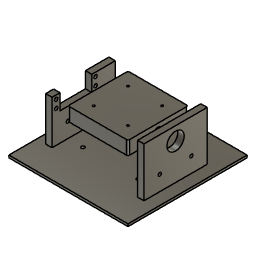
lidar_mount_prototype (Autodesk Fusion 360 design; units mm, degrees)
Autodesk Fusion 360 part; units mm, degrees
sketch "sketchBase" plane through (0, 0, 0) normal (0, 0, 1) x (1, 0, 0)
  line L0 (27.8, 27.8) -> (-27.8, 27.8) construction
  line L1 (-27.8, 27.8) -> (-27.8, -27.8) construction
  line L2 (-27.8, -27.8) -> (27.8, -27.8) construction
  line L3 (27.8, -27.8) -> (27.8, 27.8) construction
  line L4 (27.8, 27.8) -> (-27.8, -27.8) construction
  line L5 (-27.8, 27.8) -> (27.8, -27.8) construction
  line L6 (37.8, 37.8) -> (-37.8, 37.8) construction
  line L7 (-37.8, 37.8) -> (-37.8, -37.8) construction
  line L8 (-37.8, -37.8) -> (37.8, -37.8) construction
  line L9 (37.8, -37.8) -> (37.8, 37.8) construction
  line L10 (37.8, 37.8) -> (-37.8, -37.8) construction
  line L11 (-37.8, 37.8) -> (37.8, -37.8) construction
  line L12 (75, 75) -> (-75, 75)
  line L13 (-75, 75) -> (-75, -75)
  line L14 (-75, -75) -> (75, -75)
  line L15 (75, -75) -> (75, 75)
  line L16 (75, 75) -> (-75, -75) construction
  line L17 (-75, 75) -> (75, -75) construction
  line L18 (-55.8, 39.8) -> (-63.8, 39.8) construction
  line L19 (-63.8, 39.8) -> (-63.8, -39.8) construction
  line L20 (-63.8, -39.8) -> (-55.8, -39.8) construction
  line L21 (-55.8, -39.8) -> (-55.8, 39.8) construction
  line L22 (-55.8, 39.8) -> (-63.8, -39.8) construction
  line L23 (-63.8, 39.8) -> (-55.8, -39.8) construction
  line L24 (59.9, -39.8) -> (59.9, 39.8) construction
  line L25 (59.9, -39.8) -> (51.9, 39.8) construction
  line L26 (51.9, -39.8) -> (59.9, 39.8) construction
  line L27 (51.9, 39.8) -> (51.9, -39.8) construction
  line L28 (51.9, -39.8) -> (59.9, -39.8) construction
  line L29 (59.9, 39.8) -> (51.9, 39.8) construction
  line L30 (-37.8, 0) -> (-36.8, 0) construction
  line L31 (37.8, 0) -> (42.8, 0) construction
  line L32 (42.8, 0) -> (50.8, 0) construction
  line L33 (50.8, 0) -> (52.4, 0) construction
  line L34 (52.4, 0) -> (59.4, 0) construction
  line L35 (59.4, 0) -> (59.9, 0) construction
  line L36 (59.9, 0) -> (55.9, 0) construction
  line L37 (51.9, 0) -> (51.9, -19.9) construction
  line L38 (51.9, -19.9) -> (32.9, -19.9) construction
  circle A0 centre (-36.8, -19.9) radius 2 construction
  circle A1 centre (-36.8, -19.9) radius 2.1
  circle A2 centre (-36.8, 19.9) radius 2.1
  circle A3 centre (-36.8, 19.9) radius 2 construction
  circle A4 centre (32.9, -19.9) radius 2 construction
  circle A5 centre (32.9, -19.9) radius 2.1
  circle A6 centre (32.9, 19.9) radius 2 construction
  circle A7 centre (32.9, 19.9) radius 2.1
  line L39 (-36.8, 0) -> (-43.3, 0) construction
  line L40 (-43.3, 0) -> (-55.8, 0) construction
  line L41 (-55.8, 0) -> (-55.8, -19.9) construction
  line L42 (-55.8, -19.9) -> (-36.8, -19.9) construction
  point P0 (-59.8, 0)
  point P1 (55.9, 0)
  dimension "d93" = 55.6
  dimension "d94" = 55.6
  dimension "d95" = 75.6
  dimension "d96" = 75.6
  dimension "d99" = 150
  dimension "d100" = 150
  dimension "d109" = 8
  dimension "d110" = 79.6
  dimension "d307" = 1
  dimension "d344" = 5
  dimension "d345" = 8
  dimension "d346" = 1.6
  dimension "d347" = 7
  dimension "d348" = 0.5
  dimension "d349" = 4
  dimension "d350" = 19.9
  dimension "d351" = 19
  dimension "d358" = 4
  dimension "d359" = 0.1
  dimension "d362" = 0
  dimension "d363" = 39.8
  dimension "d369" = 4
  dimension "d370" = 0.1
  dimension "d373" = 0
  dimension "d374" = 39.8
  dimension "d375" = 6.5
  dimension "d376" = 12.5
  dimension "d377" = 19.9
  dimension "d378" = 19
  constraint horizontal L0
  constraint perpendicular L0 L1
  constraint parallel L0 L2
  constraint parallel L1 L3
  constraint coincident L4 origin
  constraint coincident L5 origin
  constraint horizontal L6
  constraint perpendicular L6 L7
  constraint parallel L6 L8
  constraint coincident L10 origin
  constraint coincident L11 origin
  constraint horizontal L12
  constraint perpendicular L12 L13
  constraint parallel L12 L14
  constraint parallel L13 L15
  constraint coincident L16 origin
  constraint coincident L17 origin
  constraint horizontal L18
  constraint perpendicular L18 L19
  constraint parallel L18 L20
  constraint parallel L19 L21
  constraint coincident L22 P0
  constraint coincident L23 P0
  constraint midpoint L7 L30.start
  constraint perpendicular L7 L30
  constraint midpoint L9 L31.start
  constraint perpendicular L9 L31
  constraint parallel L31 L32
  constraint parallel L32 L33
  constraint perpendicular L24 L34
  constraint parallel L34 L35
  constraint parallel L34 L36
  constraint midpoint L26 P1
  constraint coincident P1 L36.end
  constraint midpoint L27 L37.start
  constraint perpendicular L33 L37
  constraint perpendicular L27 L38
  constraint coincident L38.end A4.centre
  constraint perpendicular L7 L39
  constraint parallel L39 L40
  constraint coincident L21 L40.end
  constraint perpendicular L40 L41
  constraint perpendicular L41 L42
  constraint coincident A0.centre A1.centre
  measures "d93" distance of L1.end L2.end
  measures "d94" distance of L0.end L1.end
  measures "d95" distance of L7.end L8.end
  measures "d96" distance of L6.end L7.end
  measures "d99" distance of L13.end L14.end
  measures "d100" distance of L12.end L13.end
  measures "d109" distance of L19.end L20.end
  measures "d110" distance of L18.end L19.end
  measures "d307" distance of L30.start L30.end
  measures "d344" distance of L31.start L31.end
  measures "d345" distance of L31.end L32.end
  measures "d346" distance of L32.end L33.end
  measures "d347" distance of L33.end L34.end
  measures "d348" distance of L34.end L35.end
  measures "d349" distance of L35.end P1
  measures "d350" distance of L37.start L37.end
  measures "d351" distance of L37.end L38.end
  measures "d358" diameter of A0
  measures "d369" diameter of A4
  measures "d375" distance of L30.end L39.end
  measures "d376" distance of L39.end L40.end
  measures "d377" distance of L40.end L41.end
  measures "d378" distance of L41.end A0.centre
ref_plane "WorkPlane1" through (0, 0, 3) normal (0, 0, 1) x (1, 0, 0)
sketch "sketchSups" plane through (0, 0, 3) normal (0, 0, 1) x (1, 0, 0)
  line L0 (-55.8, 39.8) -> (-63.8, 39.8)
  line L1 (-55.8, -39.8) -> (-55.8, 39.8)
  line L2 (-63.8, 39.8) -> (-63.8, -39.8)
  line L3 (-63.8, -39.8) -> (-55.8, -39.8)
  line L4 (51.9, 39.8) -> (51.9, -39.8)
  line L5 (59.9, 39.8) -> (51.9, 39.8)
  line L6 (59.9, -39.8) -> (59.9, 39.8)
  line L7 (51.9, -39.8) -> (59.9, -39.8)
extrude "Extrude5" add sketch "sketchSups" along normal blind 55 contours L0 L1 L2 L3 makes body 1
extrude "Extrude6" add sketch "sketchSups" along normal blind 62 separate body contours L4 L5 L6 L7 makes body 2
sketch "sketchServoSup" plane through (-55.8, 0, 0) normal (1, 0, 0) x (0, 1, 0)
  line L0 (-39.8, 3) -> (39.8, 3)
  line L1 (39.8, 3) -> (39.8, 58)
  line L2 (39.8, 58) -> (-39.8, 58)
  line L3 (-39.8, 58) -> (-39.8, 3)
  line L4 (0, 58) -> (0, 48.2) construction
  line L5 (0, 48.2) -> (-9.8, 48.2) construction
  line L6 (10, 58) -> (-29.6, 58) construction
  line L7 (-29.6, 58) -> (-29.6, 38.4) construction
  line L8 (-29.6, 38.4) -> (10, 38.4) construction
  line L9 (10, 38.4) -> (10, 58) construction
  line L10 (10, 58) -> (-29.6, 38.4) construction
  line L11 (-29.6, 58) -> (10, 38.4) construction
  line L12 (-9.8, 48.2) -> (-34.55, 48.2) construction
  line L13 (-34.55, 48.2) -> (-34.55, 43.2) construction
  circle A0 centre (-34.55, 43.2) radius 2.05
  circle A1 centre (-34.55, 43.2) radius 2.15
  circle A2 centre (14.95, 43.2) radius 2.15
  circle A3 centre (14.95, 43.2) radius 2.05
  circle A4 centre (-34.55, 53.2) radius 2.15
  circle A5 centre (-34.55, 53.2) radius 2.05
  circle A6 centre (14.95, 53.2) radius 2.15
  circle A7 centre (14.95, 53.2) radius 2.05
  line L14 (0, 3) -> (0, 22) construction
  line L15 (0, 22) -> (-19.9, 22) construction
  circle A8 centre (-19.9, 22) radius 2
  circle A9 centre (-19.9, 22) radius 2.1
  circle A10 centre (19.9, 22) radius 2.1
  circle A11 centre (19.9, 22) radius 2
  line L16 (10.2, 58.2) -> (-29.8, 58.2)
  line L17 (-29.8, 58.2) -> (-29.8, 38.2)
  line L18 (-29.8, 38.2) -> (10.2, 38.2)
  line L19 (10.2, 38.2) -> (10.2, 58.2)
  point P0 (-9.8, 48.2)
  dimension "d147" = 9.8
  dimension "d148" = 9.8
  dimension "d149" = 39.6
  dimension "d150" = 19.6
  dimension "d152" = 24.75
  dimension "d153" = 5
  dimension "d154" = 4.1
  dimension "d155" = 0.1
  dimension "d158" = 49.5
  dimension "d159" = 10
  dimension "d213" = 19
  dimension "d214" = 19.9
  dimension "d215" = 4
  dimension "d216" = 0.1
  dimension "d219" = 39.8
  dimension "d220" = 0
  dimension "d380" = 0.2
  constraint midpoint L2 L4.start
  constraint perpendicular L2 L4
  constraint perpendicular L4 L5
  constraint horizontal L6
  constraint perpendicular L6 L7
  constraint parallel L6 L8
  constraint parallel L7 L9
  constraint coincident L10 P0
  constraint coincident L11 P0
  constraint coincident P0 L5.end
  constraint parallel L5 L12
  constraint perpendicular L12 L13
  constraint coincident L13.end A0.centre
  constraint midpoint L0 L14.start
  constraint perpendicular L0 L14
  constraint perpendicular L14 L15
  constraint coincident L15.end A8.centre
  measures "d147" distance of L4.start L4.end
  measures "d148" distance of L4.end P0
  measures "d149" distance of L7.end L8.end
  measures "d150" distance of L6.end L7.end
  measures "d152" distance of P0 L12.end
  measures "d153" distance of L12.end L13.end
  measures "d154" diameter of A0
  measures "d213" distance of L14.start L14.end
  measures "d214" distance of L14.end L15.end
  measures "d215" diameter of A8
sketch "sketchBearingSup" plane through (51.9, 0, 0) normal (-1, 0, 0) x (0, -1, 0)
  line L0 (-39.8, 3) -> (39.8, 3)
  line L1 (39.8, 3) -> (39.8, 65)
  line L2 (39.8, 65) -> (-39.8, 65)
  line L3 (-39.8, 65) -> (-39.8, 3)
  line L4 (0, 3) -> (0, 22) construction
  line L5 (0, 22) -> (-19.9, 22) construction
  circle A0 centre (-19.9, 22) radius 2
  circle A1 centre (-19.9, 22) radius 2.1
  circle A2 centre (19.9, 22) radius 2
  circle A3 centre (19.9, 22) radius 2.1
  line L6 (0, 3) -> (0, 48.2) construction
  circle A4 centre (0, 48.2) radius 11 construction
  circle A5 centre (0, 48.2) radius 10.85
  circle A6 centre (0, 48.2) radius 3
  line L7 (0, 3) -> (0, 22) construction
  dimension "d223" = 19.9
  dimension "d225" = 4
  dimension "d226" = 0.1
  dimension "d229" = 39.8
  dimension "d230" = 0
  dimension "d252" = 45.2
  dimension "d253" = 22
  dimension "d255" = 0.15
  dimension "d263" = 6
  dimension "d342" = 19
  constraint midpoint L0 L4.start
  constraint perpendicular L0 L4
  constraint perpendicular L4 L5
  constraint coincident L5.end A0.centre
  constraint perpendicular L0 L6
  constraint coincident L6.end A4.centre
  constraint perpendicular L5 L7
  constraint coincident L4.end L5.start
  measures "d223" distance of L4.end L5.end
  measures "d225" diameter of A0
  measures "d252" distance of L4.start L6.end
  measures "d253" diameter of A4
  measures "d263" diameter of A6
  measures "d342" distance of L4.start L4.end
ref_plane "WorkPlane6" through (0, 0, 39.7) normal (0, 0, 1) x (1, 0, 0)
sketch "sketchLidarSup" plane through (0, 0, 39.7) normal (0, 0, 1) x (1, 0, 0)
  line L0 (-37.8, 37.8) -> (-37.8, -37.8)
  line L1 (37.8, 37.8) -> (-37.8, 37.8)
  line L2 (37.8, -37.8) -> (37.8, 37.8)
  line L3 (-37.8, -37.8) -> (37.8, -37.8)
  line L4 (0, 0) -> (-21.5, 0) construction
  line L5 (-21.5, 0) -> (-21.5, -21.5) construction
  circle A0 centre (-21.5, -21.5) radius 1.25 construction
  circle A1 centre (-21.5, -21.5) radius 1.35
  circle A2 centre (21.5, -21.5) radius 1.35
  circle A3 centre (21.5, -21.5) radius 1.25 construction
  circle A4 centre (-21.5, 21.5) radius 1.35
  circle A5 centre (-21.5, 21.5) radius 1.25 construction
  circle A6 centre (21.5, 21.5) radius 1.35
  circle A7 centre (21.5, 21.5) radius 1.25 construction
  dimension "d188" = 21.5
  dimension "d189" = 21.5
  dimension "d190" = 2.5
  dimension "d191" = 0.1
  dimension "d194" = 43
  dimension "d195" = 43
  constraint coincident L4.start origin
  constraint horizontal L4
  constraint perpendicular L4 L5
  constraint coincident L5.end A0.centre
  measures "d188" distance of L4.start L4.end
  measures "d189" distance of L4.end L5.end
  measures "d190" diameter of A0
extrude "Extrude11" add sketch "sketchLidarSup" along normal blind 17 separate body makes body 3
extrude "Extrude12" cut sketch "sketchBearingSup" along normal mid plane 40 contours A0 | A1 | A2 | A3 bodies 2
extrude "Extrude13" cut sketch "sketchServoSup" along normal mid plane 40 contours A8 | A9 | A10 | A11 bodies 1
extrude "Extrude14" cut sketch "sketchServoSup" against normal blind 20 contours A0 | A1 | A2 | A3 | A4 | A5 | A6 | A7 bodies 1
extrude "Extrude23" cut sketch "sketchServoSup" against normal blind 8 contours L2 L16 L17 L19 | L2 L17 L18 L19 bodies 1
extrude "Extrude17" cut sketch "sketchBearingSup" against normal blind 20 contours A5 | A6 bodies 2
sketch "sketchTurningScrew" plane through (37.8, 0, 0) normal (1, 0, 0) x (0, 1, 0)
  line L0 (-37.8, 39.7) -> (37.8, 39.7)
  line L1 (37.8, 39.7) -> (37.8, 56.7)
  line L2 (37.8, 56.7) -> (-37.8, 56.7)
  line L3 (-37.8, 56.7) -> (-37.8, 39.7)
  line L4 (0, 39.7) -> (0, 48.2) construction
  circle A0 centre (0, 48.2) radius 4 construction
  circle A1 centre (0, 48.2) radius 4.2
  dimension "d274" = 8.5
  dimension "d317" = 8
  dimension "d318" = 0.2
  constraint midpoint L0 L4.start
  constraint perpendicular L2 L4
  constraint coincident L4.end A0.centre
  measures "d274" distance of L4.start L4.end
  measures "d317" diameter of A0
sketch "sketchNotch" plane through (-37.8, 0, 0) normal (-1, 0, 0) x (0, -1, 0)
  line L0 (-37.8, 39.7) -> (37.8, 39.7)
  line L1 (37.8, 39.7) -> (37.8, 56.7)
  line L2 (37.8, 56.7) -> (-37.8, 56.7)
  line L3 (-37.8, 56.7) -> (-37.8, 39.7)
  line L4 (0, 39.7) -> (0, 48.2) construction
  line L5 (19.15, 54.2) -> (-19.15, 54.2) construction
  line L6 (-19.15, 54.2) -> (-19.15, 42.2) construction
  line L7 (-19.15, 42.2) -> (19.15, 42.2) construction
  line L8 (19.15, 42.2) -> (19.15, 54.2) construction
  line L9 (19.15, 54.2) -> (-19.15, 42.2) construction
  line L10 (-19.15, 54.2) -> (19.15, 42.2) construction
  line L11 (19.45, 41.9) -> (19.45, 54.5)
  line L12 (19.45, 54.5) -> (-19.45, 54.5)
  line L13 (-19.45, 54.5) -> (-19.45, 41.9)
  line L14 (-19.45, 41.9) -> (19.45, 41.9)
  line L15 (0, 48.2) -> (-16.1, 48.2) construction
  circle A0 centre (-16.1, 48.2) radius 1 construction
  circle A1 centre (-16.1, 48.2) radius 1.2
  circle A2 centre (16.1, 48.2) radius 1 construction
  circle A3 centre (16.1, 48.2) radius 1.2
  point P0 (0, 48.2)
  dimension "d281" = 8.5
  dimension "d282" = 38.3
  dimension "d283" = 12
  dimension "d284" = 0.3
  dimension "d285" = 16.1
  dimension "d286" = 2
  dimension "d287" = 0.2
  dimension "d290" = 32.2
  dimension "d291" = 0
  constraint midpoint L0 L4.start
  constraint perpendicular L0 L4
  constraint horizontal L5
  constraint perpendicular L5 L6
  constraint parallel L5 L7
  constraint parallel L6 L8
  constraint coincident L9 P0
  constraint coincident L10 P0
  constraint coincident P0 L4.end
  constraint perpendicular L4 L15
  constraint coincident L15.end A0.centre
  measures "d281" distance of L4.start P0
  measures "d282" distance of L6.end L7.end
  measures "d283" distance of L5.end L6.end
  measures "d285" distance of P0 L15.end
  measures "d286" diameter of A0
extrude "Extrude20" cut sketch "sketchNotch" against normal blind 3.1 contours L11 L12 L13 L14 | A1 | A3 bodies 3
sketch "sketchNotchHoles" plane through (-34.7, 0, 0) normal (-1, 0, 0) x (0, -1, 0)
  line L0 (19.45, 41.9) -> (19.45, 54.5)
  line L1 (-19.45, 54.5) -> (-19.45, 41.9)
  circle A0 centre (-16.1, 48.2) radius 1.2
  circle A1 centre (16.1, 48.2) radius 1.2
  line L2 (-19.45, 41.9) -> (19.45, 41.9)
  line L3 (19.45, 54.5) -> (-19.45, 54.5)
extrude "Extrude21" cut sketch "sketchNotchHoles" against normal blind 10 contours A0 | A1 bodies 3
fillet "Fillet1" radius 2 4 edges at (37.8, -37.8, 48.2) (-37.8, -37.8, 48.2) (37.8, 37.8, 48.2) (-37.8, 37.8, 48.2) on bodies 3
sketch "sketchLidarSupBottom" plane through (0, 0, 39.7) normal (0, 0, -1) x (1, 0, 0)
  circle A0 centre (21.5, -21.5) radius 1.35
  circle A1 centre (-21.5, -21.5) radius 1.35
  circle A2 centre (-21.5, 21.5) radius 1.35
  circle A3 centre (21.5, 21.5) radius 1.35
  arc A4 (-37.8, -35.8) -> (-35.8, -37.8) centre (-35.8, -35.8) ccw
  line L0 (-35.8, -37.8) -> (35.8, -37.8)
  arc A5 (35.8, -37.8) -> (37.8, -35.8) centre (35.8, -35.8) ccw
  line L1 (37.8, -35.8) -> (37.8, 35.8)
  arc A6 (37.8, 35.8) -> (35.8, 37.8) centre (35.8, 35.8) ccw
  line L2 (35.8, 37.8) -> (-35.8, 37.8)
  arc A7 (-35.8, 37.8) -> (-37.8, 35.8) centre (-35.8, 35.8) ccw
  line L3 (-37.8, 35.8) -> (-37.8, -35.8)
  line L4 (21.5, -21.5) -> (-21.5, -21.5) construction
  line L5 (-21.5, -21.5) -> (-21.5, 21.5) construction
  line L6 (-21.5, 21.5) -> (21.5, 21.5) construction
  line L7 (21.5, 21.5) -> (21.5, -21.5) construction
  line L8 (24.5, -24.5) -> (-24.5, -24.5)
  line L9 (-24.5, -24.5) -> (-24.5, 24.5)
  line L10 (-24.5, 24.5) -> (24.5, 24.5)
  line L11 (24.5, 24.5) -> (24.5, -24.5)
  line L12 (24.5, 0) -> (24.5, 10.75) construction
  line L13 (24.5, 10.75) -> (16.5, 10.75)
  line L14 (16.5, 10.75) -> (16.5, -10.75)
  line L15 (16.5, -10.75) -> (24.5, -10.75)
  dimension "d331" = 10.75
  dimension "d332" = 8
  dimension "d333" = 21.5
  constraint horizontal L4
  constraint vertical L5
  constraint horizontal L6
  constraint vertical L7
  constraint coincident A2.centre L5.end
  constraint coincident A0.centre L4.start
  constraint midpoint L11 L12.start
  constraint parallel L11 L12
  constraint perpendicular L11 L13
  constraint perpendicular L13 L14
  constraint coincident L11 L15.end
  constraint perpendicular L11 L15
  measures "d331" distance of L12.start L12.end
  measures "d332" distance of L12.end L13.end
  measures "d333" distance of L13.end L14.end
extrude "Extrude25" cut sketch "sketchLidarSupBottom" against normal blind 5 contours L8 L9 L10 L11 L13 L14 L15 bodies 3
fillet "Fillet4" radius 2 8 edges at (24.5, -24.5, 42.2) (24.5, -10.75, 42.2) (16.5, -10.75, 42.2) (-24.5, -24.5, 42.2) (16.5, 10.75, 42.2) (24.5, 10.75, 42.2) (24.5, 24.5, 42.2) (-24.5, 24.5, 42.2) on bodies 3
extrude "Extrude26" cut sketch "sketchTurningScrew" against normal blind 13.7 contours A1 bodies 3
extrude "Extrude28" add sketch "sketchBase" along normal blind 3 separate body makes body 4
fillet "Fillet5" radius 0.5 10 edges at (-34.7, 19.45, 48.2) (-34.7, -19.45, 48.2) (-37.8, 19.45, 48.2) (-37.8, -19.45, 48.2) (-34.7, 0, 41.9) (-34.7, 0, 54.5) (-36.25, -19.45, 54.5) (-36.25, -19.45, 41.9) (-36.25, 19.45, 41.9) (-36.25, 19.45, 54.5) on bodies 3
sketch "servoSup" plane through (-63.8, 0, 0) normal (-1, 0, 0) x (0, -1, 0)
  line L0 (29.8, 58) -> (29.8, 38.2)
  line L1 (29.8, 38.2) -> (-10.2, 38.2)
  line L2 (-10.2, 38.2) -> (-10.2, 58)
  line L3 (-10.2, 58) -> (-39.8, 58)
  line L4 (-39.8, 58) -> (-39.8, 3)
  line L5 (-39.8, 3) -> (39.8, 3)
  line L6 (39.8, 3) -> (39.8, 58)
  line L7 (39.8, 58) -> (29.8, 58)
  circle A0 centre (-19.9, 22) radius 2.1
  circle A1 centre (19.9, 22) radius 2.1
  circle A2 centre (-14.95, 43.2) radius 2.15
  circle A3 centre (34.55, 53.2) radius 2.15
  circle A4 centre (-14.95, 53.2) radius 2.15
  circle A5 centre (34.55, 43.2) radius 2.15
  line L8 (-10.2, 58) -> (-10.2, 38.2)
  line L9 (-10.2, 38.2) -> (29.8, 38.2)
  line L10 (29.8, 38.2) -> (29.8, 58)
  line L11 (-10.2, 58) -> (-39.8, 58)
  circle A6 centre (34.55, 43.2) radius 2.15
  circle A7 centre (-14.95, 53.2) radius 2.15
  circle A8 centre (34.55, 53.2) radius 2.15
  circle A9 centre (-14.95, 43.2) radius 2.15
  circle A10 centre (19.9, 22) radius 2.1
  circle A11 centre (-19.9, 22) radius 2.1
  line L12 (-39.8, 3) -> (-39.8, 58)
  line L13 (39.8, 58) -> (29.8, 58)
  line L14 (39.8, 3) -> (39.8, 58)
  line L15 (39.8, 3) -> (-39.8, 3)
sketch "bearingSup" plane through (59.9, 0, 0) normal (1, 0, 0) x (0, 1, 0)
  circle A0 centre (0, 48.2) radius 10.85
  circle A1 centre (-19.9, 22) radius 2.1
  circle A2 centre (19.9, 22) radius 2.1
  line L0 (-39.8, 3) -> (39.8, 3)
  line L1 (39.8, 3) -> (39.8, 65)
  line L2 (39.8, 65) -> (-39.8, 65)
  line L3 (-39.8, 65) -> (-39.8, 3)
  circle A3 centre (0, 48.2) radius 10.85
  circle A4 centre (-19.9, 22) radius 2.1
  circle A5 centre (19.9, 22) radius 2.1
  line L4 (39.8, 3) -> (-39.8, 3)
  line L5 (-39.8, 3) -> (-39.8, 65)
  line L6 (39.8, 65) -> (-39.8, 65)
  line L7 (39.8, 3) -> (39.8, 65)
sketch "basePlate" plane through (0, 0, 3) normal (0, 0, 1) x (-1, 0, 0)
  circle A0 centre (36.8, 19.9) radius 2.1
  circle A1 centre (-32.9, -19.9) radius 2.1
  circle A2 centre (-32.9, 19.9) radius 2.1
  circle A3 centre (36.8, -19.9) radius 2.1
  line L0 (-75, 75) -> (-75, -75)
  line L1 (-75, -75) -> (75, -75)
  line L2 (75, -75) -> (75, 75)
  line L3 (75, 75) -> (-75, 75)
  circle A4 centre (36.8, -19.9) radius 2.1
  circle A5 centre (-32.9, 19.9) radius 2.1
  circle A6 centre (-32.9, -19.9) radius 2.1
  circle A7 centre (36.8, 19.9) radius 2.1
  line L4 (75, 75) -> (-75, 75)
  line L5 (75, -75) -> (75, 75)
  line L6 (-75, -75) -> (75, -75)
  line L7 (-75, 75) -> (-75, -75)
equation "baseWidth = 150 mm"
equation "baseLength = 150 mm"
equation "margin = 0.1 mm"
equation "plateDepth = 3 mm"
equation "lidarLength = 55.6 mm"
equation "lidarSupOffset = 10 mm"
equation "servoSupWidth = 8 mm"
equation "servoSupLengthOffset = 20 mm"
equation "servoSupHeight = 55 mm"
equation "servoLength = 39.6 mm"
equation "servoHeight = 19.6 mm"
equation "d39 = plateDepth"
equation "armToServo = 6.5 mm"
equation "servoInnerDepth = 12.5 mm"
equation "LBracketHoleDiameter = 4 mm"
equation "toLBracketHole = 19 mm"
equation "toServoShaft = 9.8 mm"
equation "d93 = lidarLength"
equation "d94 = lidarLength"
equation "d95 = lidarLength + 2 * lidarSupOffset"
equation "d96 = lidarLength + 2 * lidarSupOffset"
equation "d99 = baseWidth"
equation "d100 = baseLength"
equation "armDepth = 2 mm"
equation "d109 = servoSupWidth"
equation "d110 = servoSupLength"
equation "servoSupLength = servoLength + 2 * servoSupLengthOffset"
equation "d135 = servoSupHeight"
equation "d137 = otherSupHeight"
equation "servoHolesLength = 49.5 mm"
equation "servoHolesHeight = 10 mm"
equation "servoHolesDiameter = 4.1 mm"
equation "d147 = servoHeight / 2"
equation "d148 = toServoShaft"
equation "d149 = servoLength"
equation "d150 = servoHeight"
equation "d152 = servoHolesLength / 2"
equation "d153 = servoHolesHeight / 2"
equation "d154 = servoHolesDiameter"
equation "d155 = margin"
equation "d158 = servoHolesLength"
equation "d159 = servoHolesHeight"
equation "toArmHole = 16.1 mm"
equation "d185 = lidarSupHeight"
equation "lidarHolesLength = 43 mm"
equation "M2_5 = 2.5 mm"
equation "d188 = lidarHolesLength / 2"
equation "d189 = lidarHolesLength / 2"
equation "d190 = M2_5"
equation "d191 = margin"
equation "d194 = lidarHolesLength"
equation "d195 = lidarHolesLength"
equation "d204 = lidarSupDepth"
equation "lidarSupDepth = armHeight + 5 mm"
equation "lidarSupHeight = servoSupHeight - servoHeight / 2 - lidarSupDepth / 2"
equation "bearingInnerDiameter = 6 mm"
equation "bearingOuterDiameter = 22 mm"
equation "d213 = toLBracketHole"
equation "d214 = servoSupLength / 4"
equation "d215 = LBracketHoleDiameter"
equation "d216 = margin"
equation "d219 = servoSupLength / 2"
equation "d223 = servoSupLength / 4"
equation "d225 = LBracketHoleDiameter"
equation "d226 = margin"
equation "d229 = servoSupLength / 2"
equation "otherSupHeight = servoSupHeight + 7 mm"
equation "d252 = servoSupHeight - servoHeight / 2"
equation "d253 = bearingOuterDiameter"
equation "bearingMargin = 0.15 mm"
equation "d255 = bearingMargin"
equation "notchDepth = armDepth + 1 mm"
equation "d263 = bearingInnerDiameter"
equation "turningScrewLength = 35 mm"
equation "d274 = lidarSupDepth / 2"
equation "armLength = 38.3 mm"
equation "armHeight = 12 mm"
equation "d281 = lidarSupDepth / 2"
equation "d282 = armLength"
equation "d283 = armHeight"
equation "d284 = notchMargin"
equation "d285 = toArmHole"
equation "d286 = M2"
equation "d287 = largeMargin"
equation "d290 = 2 * toArmHole"
equation "d292 = -( notchDepth + margin )"
equation "armScrewsLength = 12 mm"
equation "d295 = -( armScrewsLength - armDepth )"
equation "filletMargin = 2 mm"
equation "d299 = filletMargin"
equation "filletTightMargin = 0.5 mm"
equation "M2 = 2 mm"
equation "d307 = notchDepth - armDepth"
equation "d309 = -servoSupWidth"
equation "turningScrewDiameter = 6 mm"
equation "bearingWidth = 7 mm"
equation "nutWidth = 8 mm"
equation "rondelleWidth = 1.6 mm"
equation "lidarSupHoleDiameter = 8 mm"
equation "lidarSupHoleDepth = 12.7 mm + 1 mm"
equation "d317 = lidarSupHoleDiameter"
equation "d318 = largeMargin"
equation "lidarScrewsLength = 16 mm"
equation "lidarSupInnerDepth = lidarScrewsLength - lidarHolesDepth"
equation "d325 = -( lidarSupDepth - lidarSupInnerDepth )"
equation "d327 = -lidarSupHoleDepth"
equation "innerRectangleOffset = 3 mm"
equation "d330 = -innerRectangleOffset"
equation "d331 = lidarHolesLength / 4"
equation "d332 = turningScrewAdditionalLength"
equation "turningScrewAdditionalLength = 8 mm"
equation "d340 = filletMargin"
equation "lidarHolesDepth = 4 mm"
equation "d342 = toLBracketHole"
equation "turningScrewOffset = 5 mm"
equation "d344 = turningScrewOffset"
equation "d345 = nutWidth"
equation "d346 = rondelleWidth"
equation "d347 = bearingWidth"
equation "d348 = ( servoSupWidth - bearingWidth ) / 2"
equation "d349 = servoSupWidth / 2"
equation "d350 = servoSupLength / 4"
equation "d351 = toLBracketHole"
equation "d358 = LBracketHoleDiameter"
equation "d359 = margin"
equation "d363 = servoSupLength / 2"
equation "d364 = plateDepth"
equation "notchMargin = 0.3 mm"
equation "d368 = filletTightMargin"
equation "d369 = LBracketHoleDiameter"
equation "d370 = margin"
equation "d374 = servoSupLength / 2"
equation "d375 = armToServo"
equation "d376 = servoInnerDepth"
equation "d377 = servoSupLength / 4"
equation "d378 = toLBracketHole"
equation "servoMargin = 0.2 mm"
equation "d380 = servoMargin"
equation "largeMargin = 0.2 mm"
named bodies: "servoSup", "bearingSup", "lidarSup", "basePlate"
